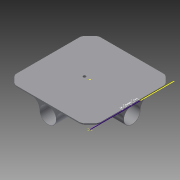
# Autodesk Inventor part: sqaureBase
Saved by Autodesk Inventor 2015 (Build 190159000, 159)
## iProperties
Created: 2015-10-11
Part Number: sqaureBase
Material: Generic
Document SubType Name: Sheet Metal
Designer: Ross
Density: 1 g/cm^3
Sheet Metal Rule: Default
Appearance: Default
Author: Ross
Autodesk Inventor part; units mm, degrees
ref_plane "YZ Plane" through (0, 0, 0) normal (1, 0, 0) x (0, 1, 0)
ref_plane "XZ Plane" through (0, 0, 0) normal (0, 1, 0) x (-1, 0, 0)
ref_plane "XY Plane" through (0, 0, 0) normal (0, 0, 1) x (1, 0, 0)
sketch "Sketch1" plane through (0, 0, 0) normal (0, 1, 0) x (-1, 0, 0)
  line L0 (75, 0) -> (75, 75)
  line L1 (75, 75) -> (-75, 75)
  line L2 (-75, 75) -> (-75, -75)
  line L3 (-75, -75) -> (75, -75)
  line L4 (75, -75) -> (75, 0)
  point P0 (0, 0)
  dimension "d0" = 75
  dimension "d1" = 75
  dimension "d2" = 150
  dimension "d3" = 150
  constraints: 10 end point, 3 perpendicular, 1 collinear, 1 point on line
  measures "d0" distance of point (0, 0) L0.start
  measures "d1" distance of L0.start L0.end
  measures "d2" distance of L0.end L1.end
  measures "d3" distance of L1.end L2.end
extrude "Extrusion1" add sketch "Sketch1" along normal blind 2
sketch "Sketch2" plane through (0, 0, 0) normal (0, -1, 0) x (1, 0, 0)
  line L0 (75, 75) -> (75, 0)
  line L1 (75, 75) -> (75, -75) projected
  line L2 (75, 0) -> (75, 15)
  line L3 (75, 0) -> (75, -15)
  point P0 (0, 0)
  dimension "d6" = 15
  dimension "d7" = 15
  constraints: 6 end point, 2 point on line, 1 midpoint
  measures "d6" distance of L0.end L2.end
  measures "d7" distance of L0.end L3.end
sketch "Sketch3" plane through (75, 0, 75) normal (1, 0, 0) x (0, 0, -1)
  line L0 (75, 0) -> (90, 0)
  line L1 (150, 0) -> (0, 0) projected
  line L2 (75, 0) -> (60, 0)
  circle A0 centre (75.0005, -15) radius 15
  circle A1 centre (75.0005, -15) radius 14.5
  line L3 (60, 0) -> (50, 0)
  arc A2 (60.0008, -14.9109) -> (50, 0) centre (44.0261, -14.8159) ccw
  arc A3 (100.001, 0) -> (90.0002, -14.9109) centre (105.9749, -14.8159) ccw
  line L4 (50, 0) -> (75, 0)
  line L5 (100.001, 0) -> (75, 0)
  dimension "d8" = 15
  dimension "d10" = 15
  dimension "d13" = 10
  constraints: 10 end point, 7 point on circle, 4 centre point, 4 point on line, 3 tangent, 2 collinear, 1 coincident
  measures "d8" distance of L0.start L0.end
  measures "d10" distance of L0.start L2.end
  measures "d13" distance of L2.end L3.end
extrude "Extrusion2" add sketch "Sketch3" against normal blind 50
pattern_circular "Circular Pattern1" count 4 over 360 about axis through (0, -10, 0) along (0, 1, 0) of "Extrusion2"
sketch "Sketch4" plane through (0, 0, 0) normal (0, 1, 0) x (-1, 0, 0)
  line L0 (-75, 75) -> (-75, 60)
  line L1 (-75, 75) -> (-75, -75) projected
  line L2 (-75, 75) -> (-60, 75)
  line L3 (-25.001, 75) -> (-75, 75) projected
  line L4 (-60, 75) -> (-75, 60)
  line L5 (-75, 60) -> (-60, 75)
  point P0 (0, 0)
  dimension "d19" = 15
  dimension "d20" = 15
  constraints: 8 end point, 4 point on line
  measures "d19" distance of L0.start L0.end
  measures "d20" distance of L0.start L2.end
extrude "Extrusion3" cut sketch "Sketch4" along normal blind 50
sketch "Sketch5" plane through (0, 2, 0) normal (0, 1, 0) x (1, 0, 0)
  line L0 (75, 75) -> (75, 60)
  line L1 (75, -60) -> (75, 75) projected
  line L2 (75, 60) -> (-75, 60)
  line L3 (75, 75) -> (-75, 75) projected
  line L4 (-75, 75) -> (-60, 75)
  line L5 (-60, 75) -> (-60, -75)
  line L6 (-75, -75) -> (-25, -75) projected
  line L7 (-75, -75) -> (-75, -60)
  line L8 (-75, 75) -> (-75, -75) projected
  line L9 (-75, -60) -> (-60, -60)
  line L10 (75, 75) -> (60, 75)
  line L11 (60, 75) -> (60, 60)
  line L12 (-60, -75) -> (-75, -60)
  line L13 (-60, 75) -> (-75, 60)
  line L14 (75, 60) -> (60, 75)
  point P0 (0, 0)
  dimension "d23" = 15
  dimension "d24" = 15
  dimension "d25" = 15
  constraints: 22 end point, 8 point on line, 3 perpendicular, 1 parallel
  measures "d23" distance of L0.start L0.end
  measures "d24" distance of L3.end L4.end
  measures "d25" distance of L0.start L10.end
extrude "Extrusion4" cut sketch "Sketch5" against normal blind 50 contours L12 L6 L7
sketch "Sketch6" plane through (0, 2, 0) normal (0, 1, 0) x (1, 0, 0)
  line L0 (75, 75) -> (75, 60)
  line L1 (75, -60) -> (75, 75) projected
  line L2 (75, 60) -> (60, 60)
  line L3 (60, 60) -> (60, 75)
  line L4 (75, 75) -> (-75, 75) projected
  line L5 (75, 60) -> (60, 75)
  point P0 (0, 0)
  dimension "d28" = 15
  dimension "d29" = 15
  constraints: 8 end point, 2 perpendicular, 2 point on line
  measures "d28" distance of L0.start L0.end
  measures "d29" distance of L0.end L2.end
extrude "Extrusion5" cut sketch "Sketch6" against normal blind 50 contours L0 L5 L4
sketch "Sketch7" plane through (0, 2, 0) normal (0, 1, 0) x (1, 0, 0)
  point P0 (0, 0)
sketch "Sketch8" plane through (0, 2, 0) normal (0, 1, 0) x (1, 0, 0)
  line L0 (-75, 75) -> (-60, 75)
  line L1 (60, 75) -> (-75, 75) projected
  line L2 (-60, 75) -> (-60, 60)
  line L3 (-60, 60) -> (-75, 60)
  line L4 (-75, 75) -> (-75, -60) projected
  line L5 (-60, 75) -> (-75, 60)
  point P0 (0, 0)
  dimension "d32" = 15
  dimension "d33" = 15
  constraints: 8 end point, 2 perpendicular, 2 point on line
  measures "d32" distance of L0.start L0.end
  measures "d33" distance of L0.end L2.end
extrude "Extrusion6" cut sketch "Sketch8" against normal blind 50 contours L0 L5 L4
fillet "Fillet1" radius 10 2 edges at (60, 1, -75) (75, 1, -60)
pattern_circular "Circular Pattern2" count 4 over 360 about axis through (0, -10, 0) along (0, 1, 0) of "Fillet1"
sketch "Sketch9" plane through (0, 2, 0) normal (0, 1, 0) x (1, 0, 0)
  circle A0 centre (-9.7626, 0) radius 2.5
  point P0 (0, 0)
  dimension "d40" = 5
  constraints: 1 centre point
  measures "d40" diameter of A0
extrude "Extrusion7" cut sketch "Sketch9" against normal blind 5
equation "\"BendRadius\" = Thickness"
equation "\"BendReliefWidth\" = Thickness"
equation "\"BendReliefDepth\" = 0.5 * Thickness"
equation "\"CornerReliefSize\" = 4 * Thickness"
equation "\"MinimumRemnant\" = 2 * Thickness"
equation "\"TransitionRadius\" = BendRadius"
equation "\"JacobiRadiusSize\" = BendRadius"
equation "\"GapSize\" = Thickness"
equation "\"Thickness\" = 3.048"
body "Solid1"
